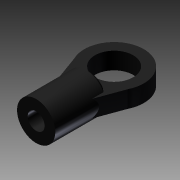
# Autodesk Inventor part: union2
Saved by Autodesk Inventor 2012 (Build 160160000, 160)
## iProperties
Created: 2013-10-01
Part Number: union2
Material: Default
Document SubType Name: Modeling
Designer: Nick
Density: 1 g/cm^3
Author: Nick
Autodesk Inventor part; units mm, degrees
ref_plane "YZ Plane" through (0, 0, 0) normal (1, 0, 0) x (0, 1, 0)
ref_plane "XZ Plane" through (0, 0, 0) normal (0, 1, 0) x (-1, 0, 0)
ref_plane "XY Plane" through (0, 0, 0) normal (0, 0, 1) x (1, 0, 0)
sketch "Sketch1" plane through (0, 0, 0) normal (0, 0, 1) x (1, 0, 0)
  circle A0 centre (0, 0) radius 2.25
  line L0 (0, 0) -> (0, -9.3774) construction
  line L1 (0, -9.3774) -> (2, -9.3774) construction
  line L2 (2, -9.3774) -> (2, -2.8723) construction
  circle A1 centre (0, 0) radius 3.5 construction
  line L3 (3.1465, -1.5328) -> (2, -4.6887)
  arc A2 (3.1465, -1.5328) -> (0, 3.5) centre (0, 0) ccw
  line L4 (-3.1465, -1.5328) -> (-2, -4.6887)
  arc A3 (0, 3.5) -> (-3.1465, -1.5328) centre (0, 0) ccw
  line L5 (2, -4.6887) -> (2, -2.8723)
  line L6 (-2, -4.6887) -> (-2, -2.8723)
  line L7 (-2, -2.8723) -> (2, -2.8723)
  dimension "d1" = 4.5
  dimension "d2" = 2
  dimension "d3" = 7
  constraints: 16 end point, 7 point on circle, 4 centre point, 3 perpendicular, 2 concentric, 2 symmetric about line, 1 coincident, 1 collinear, 1 parallel, 1 point on line, 1 vertical, 1 other
  measures "d1" diameter of A0
  measures "d2" distance of L0.end L1.end
  measures "d3" diameter of A1
extrude "Extrusion1" add sketch "Sketch1" along normal blind 2
sketch "Sketch2" plane through (-2, -2.8723, 0) normal (0, -1, 0) x (1, 0, 0)
  line L0 (4, 2) -> (0, 2) projected
  line L1 (0, 0) -> (0, 2) projected
  line L2 (0, 0) -> (4, 0) projected
  line L3 (4, 0) -> (4, 2) projected
  line L4 (0, 2) -> (4, 0) construction
  line L5 (4, 2) -> (0, 0) construction
  circle A0 centre (2, 1) radius 2.25
  point P0 (2, 0)
  dimension "d6" = 4.5
  constraints: 4 end point, 1 centre point, 1 midpoint
  measures "d6" diameter of A0
extrude "Extrusion2" add sketch "Sketch2" along normal blind 6.3 contours L3 L2 L1 L0 | A0
sketch "Sketch3" plane through (0, -9.1723, 1) normal (0, -1, 0) x (1, 0, 0)
  circle A0 centre (0, 0) radius 2.25 projected
  circle A1 centre (0, 0) radius 1
  point P0 (0, -1)
  dimension "d9" = 2
  constraints: 1 centre point, 1 coincident
  measures "d9" diameter of A1
extrude "Extrusion3" cut sketch "Sketch3" against normal blind 3 contours A1
chamfer "Chamfer1" distance 0.4 angle 45 1 edges at (0, -2.8723, -1.25)
chamfer "Chamfer2" distance 0.4 angle 45 1 edges at (0, -2.8723, 3.25)
body "Solid1"
